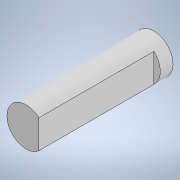
# Autodesk Inventor part: Ось мотора серии N
Saved by Autodesk Inventor 2020 (Build 240168000, 168)
## iProperties
Created: 2021-05-24
Part Number: Ось мотора серии N
Material: Типовые
Document SubType Name: Modeling
Designer: Антон
Density: 1 g/cm^3
Appearance: По умолчанию
Author: Антон
Autodesk Inventor part; units mm, degrees
ref_plane "YZ Plane" through (0, 0, 0) normal (1, 0, 0) x (0, 1, 0)
ref_plane "XZ Plane" through (0, 0, 0) normal (0, 1, 0) x (-1, 0, 0)
ref_plane "XY Plane" through (0, 0, 0) normal (0, 0, 1) x (1, 0, 0)
sketch "Эскиз1" plane through (0, 0, 0) normal (0, 0, 1) x (1, 0, 0)
  circle A0 centre (0, 0) radius 1.5
  dimension "d0" = 3
  constraints: 1 centre point, 1 coincident
  measures "d0" diameter of A0
extrude "Выдавливание1" add sketch "Эскиз1" along normal blind 10
sketch "Эскиз2" plane through (0, 0, 10) normal (0, 0, 1) x (1, 0, 0)
  line L0 (-1, -1.5) -> (1, -1.5)
  line L1 (1, -1.5) -> (1, 1.5)
  line L2 (1, 1.5) -> (-1, 1.5)
  line L3 (-1, 1.5) -> (-1, -1.5)
  circle A0 centre (0, 0) radius 1.5 projected
  line L4 (-1, -1.5) -> (1, 1.5) construction
  line L5 (1, -1.5) -> (-1, 1.5) construction
  point P0 (1, -1.118)
  point P1 (1, 1.118)
  dimension "d3" = 2
  constraints: 12 end point, 2 midpoint, 2 parallel, 1 horizontal, 1 perpendicular, 1 tangent
  measures "d3" distance of L2.end L1.end
extrude "Выдавливание2" cut sketch "Эскиз2" against normal blind 9 contours L1 A0
